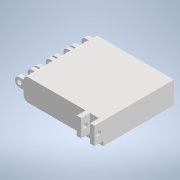
# Autodesk Inventor part: Main
Saved by Autodesk Inventor 2022 (Build 260153000, 153)
## iProperties
Created: 2022-03-12
Part Number: Main
Material: Générique
Document SubType Name: Modeling
Designer: timot
Density: 1 g/cm^3
Appearance: Par défaut
Author: timot
Autodesk Inventor part; units mm, degrees
ref_plane "YZ Plane" through (0, 0, 0) normal (1, 0, 0) x (0, 1, 0)
ref_plane "XZ Plane" through (0, 0, 0) normal (0, 1, 0) x (-1, 0, 0)
ref_plane "XY Plane" through (0, 0, 0) normal (0, 0, 1) x (1, 0, 0)
sketch "Esquisse1" plane through (0, 0, 0) normal (0, 1, 0) x (-1, 0, 0)
  line L0 (79.4884, 73.4308) -> (-10.5116, 73.4308)
  line L1 (-10.5116, 73.4308) -> (-10.5116, -6.5692)
  line L2 (-10.5116, -6.5692) -> (79.4884, -6.5692)
  line L3 (79.4884, -6.5692) -> (79.4884, 73.4308)
  point P0 (0, 0)
  dimension "d0" = 90
  dimension "d1" = 80
  constraints: 8 end point, 2 parallel, 1 horizontal, 1 perpendicular
  measures "d0" distance of L1.end L2.end
  measures "d1" distance of L0.end L1.end
extrude "Extrusion1" add sketch "Esquisse1" along normal blind 25
sketch "Esquisse6" plane through (-79.4884, 0, -6.5692) normal (-1, 0, 0) x (0, 0, 1)
  line L0 (80, 0) -> (0, 0) projected
  line L1 (40, 0) -> (40, 25)
  line L2 (0, 25) -> (90, 25) projected
  line L3 (20, 25) -> (20, 0)
  line L4 (60, 25) -> (60, 0)
  line L5 (0, 0) -> (0, 25) projected
  line L6 (80, 0) -> (80, 25) projected
  line L7 (19, 0) -> (21, 0)
  line L8 (21, 0) -> (21, 25)
  line L9 (21, 25) -> (19, 25)
  line L10 (19, 25) -> (19, 0)
  line L11 (19, 0) -> (21, 25) construction
  line L12 (21, 0) -> (19, 25) construction
  line L13 (39, 0) -> (41, 0)
  line L14 (41, 0) -> (41, 25)
  line L15 (41, 25) -> (39, 25)
  line L16 (39, 25) -> (39, 0)
  line L17 (39, 0) -> (41, 25) construction
  line L18 (41, 0) -> (39, 25) construction
  line L19 (59, 0) -> (61, 0)
  line L20 (61, 0) -> (61, 25)
  line L21 (61, 25) -> (59, 25)
  line L22 (59, 25) -> (59, 0)
  line L23 (59, 0) -> (61, 25) construction
  line L24 (61, 0) -> (59, 25) construction
  point P0 (6.5692, 0)
  point P1 (20, 12.5)
  point P2 (40, 12.5)
  point P3 (60, 12.5)
  dimension "d15" = 25
  dimension "d16" = 20
  dimension "d17" = 20
  dimension "d18" = 20
  dimension "d19" = 20
  dimension "d21" = 2
  dimension "d22" = 2
  dimension "d23" = 2
  constraints: 42 end point, 10 midpoint, 6 parallel, 6 point on line, 4 perpendicular, 3 horizontal, 2 vertical
  measures "d15" distance of L3.start L3.end
  measures "d16" distance between parallel lines of L1 L3
  measures "d17" distance between parallel lines of L1 L4
  measures "d18" distance between parallel lines of L5 L3
  measures "d19" distance between parallel lines of L6 L4
  measures "d21" distance of L9.end L8.end
  measures "d22" distance of L15.end L14.end
  measures "d23" distance of L21.end L20.end
extrude "Extrusion5" add sketch "Esquisse6" along normal blind 10 contours L0 L20 L2 L6 | L0 L14 L2 L22 | L0 L8 L2 L16 | L0 L5 L2 L10
sketch "Esquisse10" plane through (10.5116, 0, -6.5692) normal (0, 0, -1) x (-1, 0, 0)
  line L0 (90, 25) -> (100, 25) projected
  line L1 (90, 25) -> (90, 0) projected
  line L2 (100, 25) -> (90, 25)
  line L3 (90, 25) -> (90, 0)
  line L4 (90, 0) -> (100, 0)
  line L5 (100, 0) -> (100, 25)
  circle A0 centre (95, 15) radius 2.5
  line L6 (100, 0) -> (100, 25) projected
  line L7 (100, 5) -> (90, 5)
  line L8 (100, 15) -> (90, 15)
  line L9 (90, 25) -> (90, 0) projected
  line L10 (95, 15) -> (95, 25)
  point P0 (10.5116, 0)
  dimension "d26" = 5
  dimension "d40" = 5
  dimension "d41" = 10
  constraints: 14 end point, 4 point on line, 3 horizontal, 2 midpoint, 2 parallel, 1 centre point, 1 perpendicular
  measures "d26" diameter of A0
  measures "d40" distance between parallel lines of L4 L7
  measures "d41" distance between parallel lines of L7 L8
extrude "Extrusion6" cut sketch "Esquisse10" against normal blind 97 contours L10 L8 A0 | A0 L8 L10 | L8 A0
sketch "Esquisse11" plane through (-89.4884, 0, -6.5692) normal (-1, 0, 0) x (0, 0, 1)
  line L0 (70.5, 0) -> (70.5, 25)
  line L1 (80, 25) -> (61, 25) projected
  line L2 (80, 0) -> (80, 25) projected
  line L3 (80, 17.5) -> (80, 12.5) projected
  line L4 (80, 15) -> (61, 15)
  line L5 (61, 12.5) -> (61, 17.5) projected
  line L6 (75.5, 27.5) -> (65.5, 27.5)
  line L7 (65.5, 27.5) -> (65.5, 2.5)
  line L8 (65.5, 2.5) -> (75.5, 2.5)
  line L9 (75.5, 2.5) -> (75.5, 27.5)
  line L10 (75.5, 27.5) -> (65.5, 2.5) construction
  line L11 (65.5, 27.5) -> (75.5, 2.5) construction
  line L12 (61, 15) -> (0, 15)
  line L13 (0, 12.5) -> (0, 17.5) projected
  line L14 (41, 0) -> (59, 0) projected
  line L15 (50, 0) -> (50, 25)
  line L16 (59, 25) -> (41, 25) projected
  line L17 (21, 0) -> (39, 0) projected
  line L18 (30, 0) -> (30, 25)
  line L19 (19, 25) -> (0, 25) projected
  line L20 (9.5, 25) -> (9.5, 0)
  line L21 (0, 0) -> (19, 0) projected
  line L22 (55, 25) -> (45, 25)
  line L23 (45, 25) -> (45, 0)
  line L24 (45, 0) -> (55, 0)
  line L25 (55, 0) -> (55, 25)
  line L26 (55, 25) -> (45, 0) construction
  line L27 (45, 25) -> (55, 0) construction
  line L28 (35, 25) -> (25, 25)
  line L29 (25, 25) -> (25, 0)
  line L30 (25, 0) -> (35, 0)
  line L31 (35, 0) -> (35, 25)
  line L32 (35, 25) -> (25, 0) construction
  line L33 (25, 25) -> (35, 0) construction
  line L34 (14.5, 25) -> (4.5, 25)
  line L35 (4.5, 25) -> (4.5, 0)
  line L36 (4.5, 0) -> (14.5, 0)
  line L37 (14.5, 0) -> (14.5, 25)
  line L38 (14.5, 25) -> (4.5, 0) construction
  line L39 (4.5, 25) -> (14.5, 0) construction
  point P0 (6.5692, 0)
  point P1 (70.5, 15)
  point P2 (50, 12.5)
  point P3 (30, 12.5)
  point P4 (9.5, 12.5)
  point P5 (4.5, 25)
  point P6 (65.5, 25)
  point P7 (75.5, 25)
  dimension "d29" = 9.5
  dimension "d30" = 10
  dimension "d31" = 10
  dimension "d32" = 10
  dimension "d33" = 10
  constraints: 60 end point, 21 midpoint, 8 parallel, 4 horizontal, 4 perpendicular, 3 point on line, 2 vertical
  measures "d29" distance between parallel lines of L2 L0
  measures "d30" distance between parallel lines of L9 L7
  measures "d31" distance of L24.end L23.end
  measures "d32" distance of L30.end L29.end
  measures "d33" distance of L36.end L35.end
extrude "Extrusion7" cut sketch "Esquisse11" against normal blind 10 contours L8 L7 L4 L0 | L0 L4 L9 L8 | L4 L7 L1 L0 | L0 L1 L9 L4 | L25 L14 L15 L12 | L12 L15 L16 L25 | L15 L14 L23 L12 | L12 L23 L16 L15 | L31 L17 L18 L12 | L12 L18 L28 L31 | L18 L17 L29 L12 | L12 L29 L28 L18 | L37 L21 L20 L12 | L12 L20 L19 L37 | L20 L21 L35 L12 | L12 L35 L19 L20
ref_plane "Plan de construction3" through (-9.4884, 5, 73.4308) normal (0, 0, 1) x (1, 0, 0)
sketch "Esquisse13" plane through (-9.4884, 5, 73.4308) normal (0, 0, 1) x (1, 0, 0)
  line L0 (-70, 20) -> (-70, -5) projected
  line L1 (-70, 5) -> (-70, 15)
  line L2 (-70, 20) -> (-80, 20) projected
  line L3 (-70, 15) -> (-80, 15)
  line L4 (-80, 15) -> (-80, 20)
  line L5 (-80, 20) -> (-70, 20)
  line L6 (-70, 20) -> (-70, 15)
  line L7 (-70, -5) -> (-80, -5) projected
  line L8 (-70, 5) -> (-80, 5)
  line L9 (-80, 5) -> (-80, -5)
  line L10 (-80, -5) -> (-70, -5)
  line L11 (-70, -5) -> (-70, 5)
  circle A0 centre (-75, 10) radius 2.5 projected
  point P0 (9.4884, -5)
  dimension "d42" = 5
  constraints: 18 end point, 4 parallel, 2 horizontal, 2 perpendicular, 2 point on line, 1 collinear
  measures "d42" distance of L3.end L2.end
extrude "Extrusion8" cut sketch "Esquisse13" against normal blind 85.75 contours L0 L3 L4 L2 | L0 L7 L9 L8
fillet "Congé3" radius 5 2 edges at (-79.4884, 25, 33.4308) (-79.4884, 0, 33.4308)
sketch "Esquisse16" plane through (10.5116, 0, 73.4308) normal (0, 0, 1) x (1, 0, 0)
  line L0 (0, 25) -> (-85, 25) projected
  line L1 (0, 0) -> (0, 25) projected
  line L2 (-6, 25) -> (0, 17)
  line L3 (0, 17) -> (-16, 5)
  line L4 (-16, 5) -> (-22, 13)
  line L5 (-22, 13) -> (-6, 25)
  line L6 (-6, 25) -> (0, 17)
  line L7 (0, 17) -> (-4, 14)
  line L8 (-4, 14) -> (-10, 22)
  line L9 (-10, 22) -> (-6, 25)
  line L10 (-22, 13) -> (-16, 5)
  line L11 (-16, 5) -> (-12, 8)
  line L12 (-12, 8) -> (-18, 16)
  line L13 (-18, 16) -> (-22, 13)
  point P0 (-4, 14)
  dimension "d47" = 20
  dimension "d48" = 6
  dimension "d49" = 8
  dimension "d50" = 5
  dimension "d51" = 5
  constraints: 24 end point, 6 parallel, 5 perpendicular, 2 point on line
  measures "d47" distance of L2.end L3.end
  measures "d48" horizontal distance of L2.start L2.end
  measures "d49" vertical distance of L2.start L2.end
  measures "d50" distance of L2.end L7.end
  measures "d51" distance of L11.end L3.end
extrude "Extrusion9" add sketch "Esquisse16" along normal blind 10 contours L2 L3 L8 L5 | L12 L3 L4 L5
sketch "Esquisse18" plane through (4.5116, 25, 83.4308) normal (0.8, 0.6, 0) x (0, 0, -1)
  line L0 (10, -10) -> (0, -10) projected
  line L1 (5, -10) -> (5, 0)
  line L2 (10, 0) -> (0, 0) projected
  circle A0 centre (5, -5) radius 2.5
  point P0 (83.4308, -17.2931)
  dimension "d54" = 5
  constraints: 3 midpoint, 2 end point, 1 centre point
  measures "d54" diameter of A0
extrude "Extrusion10" cut sketch "Esquisse18" against normal blind 20
